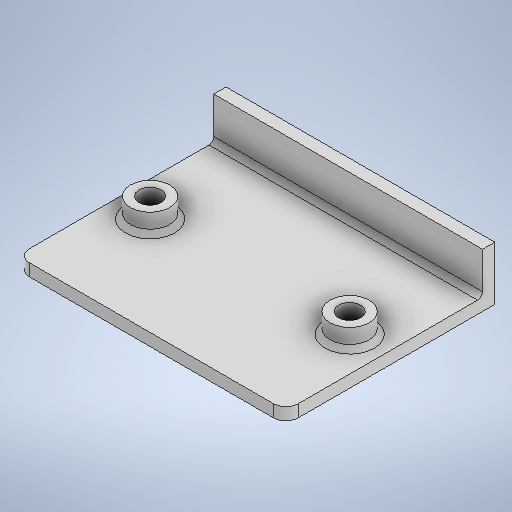
# Autodesk Inventor part: small_backplate
Saved by Autodesk Inventor 2025.2 (Build 292293000, 293)
## iProperties
Created: 2025-03-30
Part Number: small_backplate
Material: Generic
Document SubType Name: Modeling
Designer: osmon
Density: 1 g/cm^3
Appearance: Default
Author: osmon
Autodesk Inventor part; units mm, degrees
ref_plane "YZ Plane" through (0, 0, 0) normal (1, 0, 0) x (0, 1, 0)
ref_plane "XZ Plane" through (0, 0, 0) normal (0, 1, 0) x (-1, 0, 0)
ref_plane "XY Plane" through (0, 0, 0) normal (0, 0, 1) x (1, 0, 0)
sketch "Sketch1" plane through (0, 0, 0) normal (0, 1, 0) x (-1, 0, 0)
  line L0 (0, 0) -> (-54.8, 0)
  line L1 (-54.8, 0) -> (-54.8, -42.6)
  line L2 (-54.8, -42.6) -> (0, -42.6)
  line L3 (0, -42.6) -> (0, 0)
  dimension "d0" = 54.8
  dimension "d1" = 42.6
  constraints: 8 end point, 2 parallel, 1 horizontal, 1 perpendicular
  measures "d0" distance of L2.end L1.end
  measures "d1" distance of L1.end L0.end
extrude "Extrusion1" add sketch "Sketch1" along normal blind 2.5
sketch "Sketch2" plane through (0, 2.5, 0) normal (0, 1, 0) x (1, 0, 0)
  line L0 (54.8, 0) -> (54.8, 42.6) projected
  line L1 (54.8, 42.6) -> (0, 42.6) projected
  line L2 (0, 42.6) -> (0, 0) projected
  line L3 (0, 0) -> (54.8, 0) projected
  line L4 (0, 42.6) -> (54.8, 42.6)
  line L5 (54.8, 42.6) -> (54.8, 40.1)
  line L6 (54.8, 40.1) -> (0, 40.1)
  line L7 (0, 40.1) -> (0, 42.6)
  dimension "d4" = 2.5
  constraints: 8 end point, 2 parallel, 1 horizontal, 1 perpendicular, 1 point on line
  measures "d4" distance of L4.end L5.end
extrude "Extrusion2" add sketch "Sketch2" along normal blind 8.5 contours L6 L2 L1 L0
sketch "Sketch3" plane through (0, 2.5, 0) normal (0, 1, 0) x (1, 0, 0)
  line L0 (54.8, 40.1) -> (0, 40.1) projected
  line L1 (0, 40.1) -> (0, 0) projected
  line L2 (0, 0) -> (54.8, 0) projected
  line L3 (54.8, 0) -> (54.8, 40.1) projected
  circle A0 centre (7.05, 20.05) radius 4
  circle A1 centre (47.75, 20.05) radius 4
  dimension "d7" = 8
  dimension "d8" = 8
  dimension "d9" = 7.05
  dimension "d10" = 7.05
  dimension "d11" = 20.05
  dimension "d12" = 20.05
  constraints: 2 centre point
  measures "d7" diameter of A0
  measures "d8" diameter of A1
  measures "d9" distance from line of A0.centre L1
  measures "d10" distance from line of L3 A1.centre
  measures "d11" distance from line of L2 A0.centre
  measures "d12" distance from line of L2 A1.centre
extrude "Extrusion3" cut sketch "Sketch3" against normal blind 0.5 contours A0 | A1
sketch "Sketch4" plane through (7.05, 2, -20.05) normal (0, 1, 0) x (1, 0, 0)
  circle A0 centre (0, 0) radius 4 projected
  circle A1 centre (0, 0) radius 4
  circle A2 centre (40.7, 0) radius 4 projected
  circle A3 centre (40.7, 0) radius 4
  point P0 (-7.05, -20.05)
  dimension "d15" = 8
  dimension "d16" = 8
  constraints: 2 centre point, 2 coincident
  measures "d15" diameter of A1
  measures "d16" diameter of A3
extrude "Extrusion4" add sketch "Sketch4" along normal blind 4.5
sketch "Sketch5" plane through (7.05, 6.5, -20.05) normal (0, 1, 0) x (1, 0, 0)
  circle A0 centre (0, 0) radius 4 projected
  circle A1 centre (0, 0) radius 2.25
  circle A2 centre (40.7, 0) radius 4 projected
  circle A3 centre (40.7, 0) radius 2.25
  point P0 (-7.05, -20.05)
  dimension "d19" = 4.5
  dimension "d20" = 4.5
  constraints: 2 centre point, 2 coincident
  measures "d19" diameter of A1
  measures "d20" diameter of A3
extrude "Extrusion5" cut sketch "Sketch5" against normal blind 4.2 contours A1 | A3
chamfer "Chamfer1" distance 1 angle 45 2 edges at (3.05, 2.5, -20.05) (43.75, 2.5, -20.05)
fillet "Fillet1" radius 2.5 2 edges at (0, 1.25, 0) (54.8, 1.25, 0)
fillet "Fillet2" radius 1 1 edges at (27.4, 2.5, -40.1)
body "Solid1"
